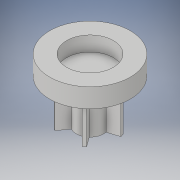
# Autodesk Inventor part: eje rodaje b
Saved by Autodesk Inventor 2019 (Build 230136000, 136)
## iProperties
Created: 2019-12-14
Part Number: eje rodaje b
Material: Generic
Document SubType Name: Modeling
Designer: HP POWER
Density: 1 g/cm^3
Appearance: Default
Author: HP POWER
Autodesk Inventor part; units mm, degrees
ref_plane "YZ Plane" through (0, 0, 0) normal (1, 0, 0) x (0, 1, 0)
ref_plane "XZ Plane" through (0, 0, 0) normal (0, 1, 0) x (-1, 0, 0)
ref_plane "XY Plane" through (0, 0, 0) normal (0, 0, 1) x (1, 0, 0)
sketch "Sketch1" plane through (0, 0, 0) normal (0, 1, 0) x (-1, 0, 0)
  circle A0 centre (0, 0) radius 4.425
  line L0 (-11.1809, -4.4215) -> (-11.6444, -2.9949)
  line L1 (-11.6444, -2.9949) -> (-6.3005, -1.2586)
  arc A1 (-4.3575, 4.7216) -> (-6.3005, -1.2586) centre (0, 0) ccw
  line L2 (-4.3575, 4.7216) -> (-7.6602, 9.2674)
  line L3 (-7.6602, 9.2674) -> (-6.4467, 10.149)
  line L4 (-6.4467, 10.149) -> (-3.1439, 5.6032)
  arc A2 (3.1439, 5.6032) -> (-3.1439, 5.6032) centre (0, 0) ccw
  line L5 (3.1439, 5.6032) -> (6.4467, 10.149)
  line L6 (6.4467, 10.149) -> (7.6602, 9.2674)
  line L7 (7.6602, 9.2674) -> (4.3575, 4.7216)
  arc A3 (6.3005, -1.2586) -> (4.3575, 4.7216) centre (0, 0) ccw
  line L8 (6.3005, -1.2586) -> (11.6444, -2.9949)
  line L9 (11.6444, -2.9949) -> (11.1809, -4.4215)
  line L10 (11.1809, -4.4215) -> (5.837, -2.6852)
  arc A4 (0.75, -6.3811) -> (5.837, -2.6852) centre (0, 0) ccw
  line L11 (0.75, -6.3811) -> (0.75, -12)
  line L12 (0.75, -12) -> (-0.75, -12)
  line L13 (-0.75, -12) -> (-0.75, -6.3811)
  arc A5 (-5.837, -2.6852) -> (-0.75, -6.3811) centre (0, 0) ccw
  line L14 (-5.837, -2.6852) -> (-11.1809, -4.4215)
  constraints: 30 end point, 10 point on circle, 6 centre point
extrude "Extrusion1" add sketch "Sketch1" along normal blind 21
sketch "Sketch2" plane through (0, 21, 0) normal (0, 1, 0) x (1, 0, 0)
  circle A0 centre (0, 0) radius 11.01
  circle A1 centre (0, 0) radius 19
  dimension "d2" = 38
  constraints: 2 centre point, 1 coincident
  measures "d2" diameter of A1
extrude "Extrusion2" add sketch "Sketch2" along normal blind 8.5
sketch "Sketch3" plane through (0, 21, 0) normal (0, 1, 0) x (1, 0, 0)
  circle A0 centre (0, 0) radius 11.01
  constraints: 1 centre point, 1 coincident
extrude "Extrusion3" add sketch "Sketch3" along normal blind 1.5
sketch "Sketch4" plane through (0, 21, 0) normal (0, -1, 0) x (1, 0, 0)
  circle A0 centre (0, 0) radius 19
  dimension "d7" = 38
  constraints: 1 centre point, 1 coincident
  measures "d7" diameter of A0
extrude "Extrusion4" add sketch "Sketch4" along normal blind 0.5
body "Solid1"
